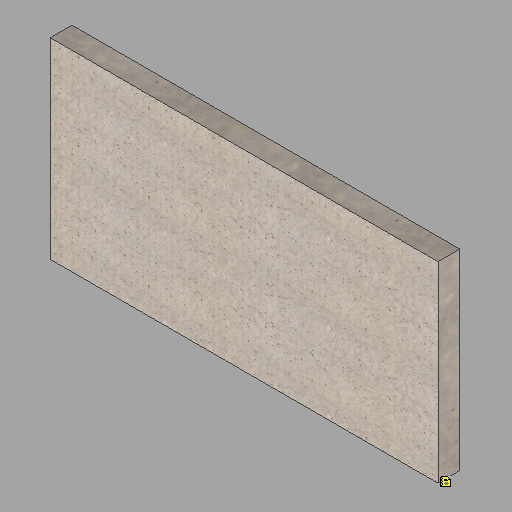
# Autodesk Inventor part: Retaining&exterior ST-2
Saved by Autodesk Inventor 2022.2 (Build 262287010, 287A)
## iProperties
Created: 2021-10-21
Part Number: Retaining&exterior ST-2
Material: Limestone
Document SubType Name: Modeling
Designer: awelt
Density: 2.6 g/cm^3
Appearance: Kasota Gray
Mass: 53504.3 g
Surface Area: 9475.99 cm^2
Volume: 20578.6 cm^3
TEST: 0.0
Author: awelt
Autodesk Inventor part; units mm, degrees
ref_plane "YZ Plane" through (0, 0, 0) normal (1, 0, 0) x (0, 1, 0)
ref_plane "XZ Plane" through (0, 0, 0) normal (0, 1, 0) x (-1, 0, 0)
ref_plane "XY Plane" through (0, 0, 0) normal (0, 0, 1) x (1, 0, 0)
sketch "Sketch1" plane through (0, 0, 0) normal (0, 1, 0) x (-1, 0, 0)
  line L0 (452.4375, -223.8375) -> (-452.4375, -223.8375)
  line L1 (-452.4375, -223.8375) -> (-452.4375, 223.8375)
  line L2 (-452.4375, 223.8375) -> (452.4375, 223.8375)
  line L3 (452.4375, 223.8375) -> (452.4375, -223.8375)
  line L4 (452.4375, -223.8375) -> (-452.4375, 223.8375) construction
  line L5 (-452.4375, -223.8375) -> (452.4375, 223.8375) construction
  point P0 (0, 0)
  dimension "d0" = 904.875
  dimension "d1" = 447.675
  constraints: 12 end point, 2 midpoint, 2 parallel, 1 horizontal, 1 perpendicular
  measures "d0" distance of L1.end L2.end
  measures "d1" distance of L0.end L1.end
extrude "Extrusion1" add sketch "Sketch1" along normal blind 50.8
sketch "Sketch2" plane through (-452.4375, 0, -223.8375) normal (-1, 0, 0) x (0, 0, 1)
  line L0 (0, 0) -> (0, 50.8) projected
  line L1 (0, 0) -> (0, 50.8) projected
  line L2 (0, 30.1625) -> (31.75, 30.1625)
  line L3 (31.75, 30.1625) -> (31.75, 20.6375)
  line L4 (31.75, 20.6375) -> (0, 20.6375)
  line L5 (0, 20.6375) -> (0, 30.1625)
  line L6 (0, 25.4) -> (53.4629, 25.4) construction
  line L7 (223.8375, 0) -> (223.8375, 50.8) construction
  line L8 (447.675, 50.8) -> (0, 50.8) construction
  line L9 (447.675, 30.1625) -> (415.925, 30.1625)
  line L10 (415.925, 30.1625) -> (415.925, 20.6375)
  line L11 (415.925, 20.6375) -> (447.675, 20.6375)
  line L12 (447.675, 20.6375) -> (447.675, 30.1625)
  dimension "d4" = 31.75
  dimension "d5" = 9.525
  constraints: 20 end point, 4 symmetric about line, 2 horizontal, 2 midpoint, 2 parallel, 1 perpendicular, 1 point on line, 1 other
  measures "d4" distance of L3.end L4.end
  measures "d5" distance of L2.end L3.end
extrude "Extrusion2" [suppressed]
body "Solid1"
